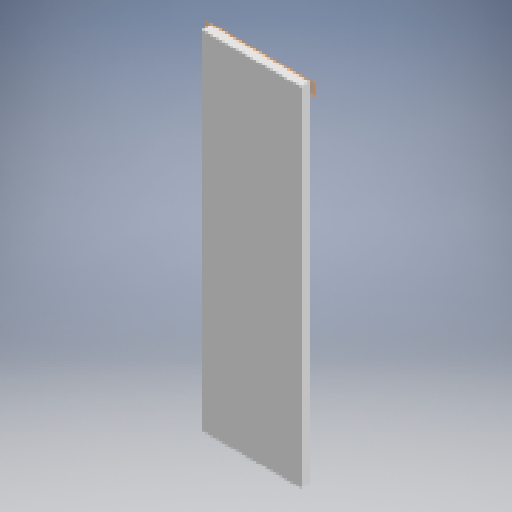
# Autodesk Inventor part: TOP SH
Saved by Autodesk Inventor 2025.2 (Build 292293000, 293)
## iProperties
Created: 2025-01-27
Part Number: TOP SH
Material: Generic
Document SubType Name: Modeling
Designer: Anna
Density: 1 g/cm^3
Appearance: Default
Author: Anna
Autodesk Inventor part; units mm, degrees
ref_plane "YZ Plane" through (0, 0, 0) normal (1, 0, 0) x (0, 1, 0)
ref_plane "XZ Plane" through (0, 0, 0) normal (0, 1, 0) x (-1, 0, 0)
ref_plane "XY Plane" through (0, 0, 0) normal (0, 0, 1) x (1, 0, 0)
ref_plane "Work Plane1" through (0, 0, 0) normal (0, 0, 1) x (1, 0, 0)
sketch "Sketch1" plane through (0, 0, 0) normal (0, 0, 1) x (1, 0, 0)
  line L0 (-7.6112, 1918.1) -> (271.7888, 1918.1) projected
  line L1 (-7.6112, 940.2) -> (271.7888, 940.2) projected
  line L2 (271.7888, 1918.1) -> (271.7888, 940.2)
  line L3 (-7.6112, 940.2) -> (-7.6112, 1918.1)
  point P0 (0, 0)
  constraints: 4 end point, 1 perpendicular, 1 vertical
extrude "Extrusion1" add sketch "Sketch1" along normal blind 25.4
body "Solid1"
